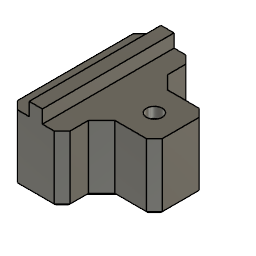
tripple leg (Autodesk Fusion 360 design; units mm, degrees)
Autodesk Fusion 360 part; units mm, degrees
sketch "Szkic1" plane through (0, 0, 0) normal (0, 0, 1) x (1, 0, 0)
  line L0 (-20, 25) -> (-20, -25)
  line L1 (-20, -25) -> (0, -25)
  line L2 (0, -25) -> (0, 25)
  line L3 (0, 25) -> (-20, 25)
  line L4 (0, 10) -> (0, -10)
  line L5 (0, -10) -> (20, -10)
  line L6 (20, -10) -> (20, 10)
  line L7 (20, 10) -> (0, 10)
  circle A0 centre (10, 0) radius 3
  circle A1 centre (10, 0) radius 5.5
  line L8 (-12.5, 25) -> (-7.5, 25)
  line L9 (-7.5, 25) -> (-7.5, -25)
  line L10 (-7.5, -25) -> (-12.5, -25)
  line L11 (-12.5, -25) -> (-12.5, 25)
  dimension "d1" = 6
  dimension "d2" = 11
  constraint perpendicular L0 L1
  constraint parallel L0 L2
  constraint parallel L1 L3
  constraint vertical L0
  constraint perpendicular L4 L5
  constraint parallel L4 L6
  constraint parallel L5 L7
  constraint coincident L2 L4.end
  constraint parallel L2 L4
  constraint concentric A0 A1
  constraint perpendicular L8 L9
  constraint parallel L8 L10
  constraint parallel L9 L11
  constraint coincident L3 L8.end
  constraint coincident L3 L8.start
  measures "d1" diameter of A0
  measures "d2" diameter of A1
extrude "Wyciągnięcie proste1" add sketch "Szkic1" against normal blind 25 contours L0 L1 L3 L11 | L1 L3 L8 L9 L10 L11 | L1 L2 L3 L4 L9 | L2 L4 L5 L6 L7
extrude "Wyciągnięcie proste2" add sketch "Szkic1" against normal blind 4.2 contours A0 | A1
extrude "Wyciągnięcie proste3" cut sketch "Szkic1" against normal blind 4 contours A0
extrude "Wyciągnięcie proste4" add sketch "Szkic1" along normal blind 5 contours L1 L3 L8 L9 L10 L11
chamfer "Fazowanie1" distance 5 angle 45 1 edges at (0, -10, -12.5)
chamfer "Fazowanie2" distance 5 angle 45 1 edges at (0, 10, -12.5)
chamfer "Fazowanie3" distance 3 angle 45 6 edges at (20, 10, -12.5) (20, -10, -12.5) (0, 25, -12.5) (-20, 25, -12.5) (-20, -25, -12.5) (0, -25, -12.5)
chamfer "Fazowanie4" distance 1 angle 45 1 faces at (-11.8333, 0, -25)
delete_face "Usuń powierzchnię1" 1 faces at (16.159, -0.3074, -24.6667)
